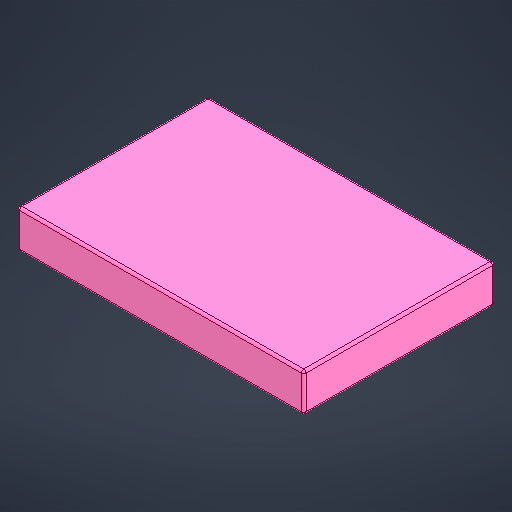
# Autodesk Inventor part: plate
Saved by Autodesk Inventor 2026 (Build 300175000, 175)
## iProperties
Created: 2025-04-21
Part Number: plate
Material: Generic
Document SubType Name: Modeling
Designer: Paul Juschitz
Density: 1 g/cm^3
Appearance: Pink
Author: Paul Juschitz
Autodesk Inventor part; units mm, degrees
ref_plane "YZ Plane" through (0, 0, 0) normal (1, 0, 0) x (0, 1, 0)
ref_plane "XZ Plane" through (0, 0, 0) normal (0, 1, 0) x (-1, 0, 0)
ref_plane "XY Plane" through (0, 0, 0) normal (0, 0, 1) x (1, 0, 0)
sketch "Sketch1" plane through (0, 0, 0) normal (0, 1, 0) x (-1, 0, 0)
  line L0 (30, 20) -> (-30, 20)
  line L1 (-30, 20) -> (-30, -20)
  line L2 (-30, -20) -> (30, -20)
  line L3 (30, -20) -> (30, 20)
  line L4 (30, 20) -> (-30, -20) construction
  line L5 (-30, 20) -> (30, -20) construction
  point P0 (0, 0)
  dimension "d0" = 60
  dimension "d1" = 40
  constraints: 12 end point, 2 midpoint, 2 parallel, 1 horizontal, 1 perpendicular
  measures "d0" distance of L1.end L2.end
  measures "d1" distance of L0.end L1.end
extrude "Extrusion1" add sketch "Sketch1" along normal blind 8
shell "Shell1" thickness 1.6 removed faces 1 at (10, 0, 6.6667)
sketch "Sketch3" plane through (-28.4, 6.4, 18.4) normal (0, -1, 0) x (1, 0, 0)
  circle A0 centre (27.5, -10.445) radius 1.5 projected
  circle A1 centre (40.4, -10.445) radius 1.5 projected
  circle A2 centre (40.4, -26.355) radius 1.5 projected
  circle A3 centre (27.5, -26.355) radius 1.5 projected
  line L0 (18.45, -4.4) -> (18.45, -32.4) projected
  line L1 (18.45, -32.4) -> (49.45, -32.4) projected
  line L2 (49.45, -32.4) -> (49.45, -4.4) projected
  line L3 (49.45, -4.4) -> (18.45, -4.4) projected
  circle A4 centre (40.4, -10.445) radius 1.5 projected
  circle A5 centre (27.5, -10.445) radius 1.5 projected
  circle A6 centre (27.5, -26.355) radius 1.5 projected
  circle A7 centre (40.4, -26.355) radius 1.5 projected
  point P0 (28.4, -18.4)
extrude "Extrusion3" add sketch "Sketch3" along normal blind 4
fillet "Fillet1" radius 0.5 36 edges at (0, 8, 20) (-30, 8, 0) (-30, 4, 20) (-30, 0, 0) (0, 0, 20) (30, 4, 20) (-30, 4, -20) (0, 0, -20) (0, 8, -20) (30, 4, -20) (30, 8, 0) (28.4, 0, 0) (30, 0, 0) (21.05, 4.4, -14) (-9.95, 4.4, -14) (-9.95, 4.4, 14) (21.05, 4.4, 14) (0, 0, 18.4) (0, 0, -18.4) (-28.4, 0, 0) (-9.95, 2.4, 0) (5.55, 2.4, -14) (21.05, 2.4, 0) (5.55, 2.4, 14) (10.5, 2.4, 7.955) (10.5, 2.4, -7.955) (-2.4, 2.4, -7.955) (-2.4, 2.4, 7.955) (28.4, 6.4, 0) (0, 6.4, -18.4) (0, 6.4, 18.4) (-28.4, 6.4, 0) (-9.95, 6.4, 0) (5.55, 6.4, 14) (21.05, 6.4, 0) (5.55, 6.4, -14)
equation "\"d0\" = plate_depth"
equation "\"d1\" = plate_width"
equation "\"plate_width\" = 40"
equation "\"plate_depth\" = 60"
body "Solid1"
